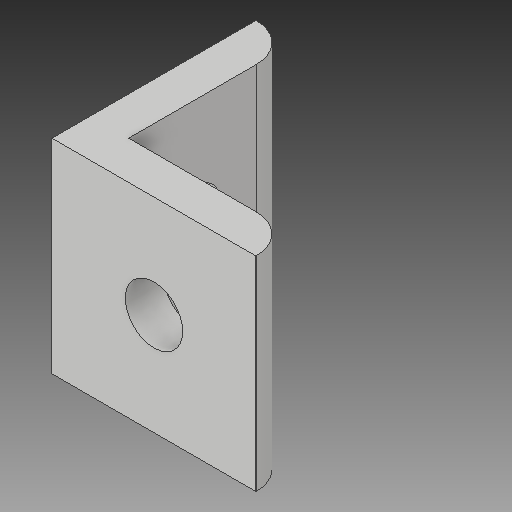
# Autodesk Inventor part: 8020_CornerBracket
Saved by Autodesk Inventor 2019 (Build 230136000, 136)
## iProperties
Created: 2018-10-13
Part Number: 8020_CornerBracket
Material: Generic
Document SubType Name: Modeling
Density: 1 g/cm^3
Appearance: Default
Title: 2-Hole Inside Corner Bracket
Autodesk Inventor part; units mm, degrees
ref_plane "YZ Plane" through (0, 0, 0) normal (1, 0, 0) x (0, 1, 0)
ref_plane "XZ Plane" through (0, 0, 0) normal (0, 1, 0) x (-1, 0, 0)
ref_plane "XY Plane" through (0, 0, 0) normal (0, 0, 1) x (1, 0, 0)
sketch "Sketch1" plane through (0, 0, 0) normal (0, 0, 1) x (1, 0, 0)
  line L0 (0, 0) -> (25.4, 0)
  line L1 (25.4, 0) -> (25.4, 25.4)
  line L2 (25.4, 25.4) -> (0, 25.4)
  line L3 (0, 25.4) -> (0, 0)
  circle A0 centre (12.7, 12.7) radius 3.5687
  dimension "d0" = 25.4
  dimension "d1" = 25.4
  dimension "d2" = 7.1374
  constraints: 8 end point, 2 parallel, 1 centre point, 1 horizontal, 1 perpendicular
  measures "d0" distance of L1.end L2.end
  measures "d1" distance of L0.end L1.end
  measures "d2" diameter of A0
extrude "Extrusion1" add sketch "Sketch1" along normal blind 4.7752
sketch "Sketch2" plane through (0, 0, 4.7752) normal (0, 0, 1) x (1, 0, 0)
  line L0 (25.4, 25.4) -> (0, 25.4) projected
  line L1 (0, 0) -> (4.7752, 0)
  line L2 (4.7752, 0) -> (4.7752, 25.4)
  line L3 (4.7752, 25.4) -> (0, 25.4)
  line L4 (0, 25.4) -> (0, 0)
  dimension "d5" = 4.7752
  constraints: 8 end point, 2 parallel, 1 horizontal, 1 perpendicular, 1 point on line
  measures "d5" distance of L1.start L1.end
extrude "Extrusion2" add sketch "Sketch2" against normal blind 25.4
sketch "Sketch3" plane through (4.7752, 0, 0) normal (1, 0, 0) x (0, 0, -1)
  line L0 (20.6248, 25.4) -> (20.6248, 0) projected
  circle A0 centre (7.9248, 12.7) radius 3.5687
  point P0 (0, 0)
  dimension "d9" = 7.1374
  constraints: 1 centre point
  measures "d9" diameter of A0
extrude "Extrusion3" cut sketch "Sketch3" against normal up to next
fillet "Fillet1" radius 4.7625 1 edges at (4.7752, 12.7, -20.6248)
fillet "Fillet2" radius 4.7625 1 edges at (25.4, 12.7, 0)
body "Solid1"
